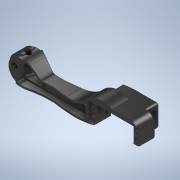
# Autodesk Inventor part: Perna_Esq_v2
Saved by Autodesk Inventor 2020 (Build 240168000, 168)
## iProperties
Created: 2021-05-05
Part Number: Perna_Esq_v2
Material: Plástico PC/ABS
Document SubType Name: Modeling
Designer: JCarlos
Density: 0.357273 g/cm^3
Appearance: Brilhosa - Preta
Mass: 11.0477 g
Surface Area: 184.649 cm^2
Volume: 30.9223 cm^3
Author: JCarlos
Autodesk Inventor part; units mm, degrees
sketch "Esboço1" plane through (0, 0, 0) normal (0, 0, 1) x (1, 0, 0)
  line L0 (97.4332, 6) -> (97.4332, -6)
  line L1 (16.7086, -15) -> (-37.5668, -15)
  line L2 (-37.286, -11) -> (-21.0787, -11)
  line L3 (-18.1298, -3.8807) -> (-30.0859, 8.0754)
  line L4 (-26.9602, 10.6066) -> (-17.8181, 1.4645)
  line L5 (-14.2825, 0) -> (14.2825, 0)
  arc A0 (67.4332, 15) -> (35.9332, 7.5) centre (56.0954, -7.2813) ccw
  arc A1 (14.2825, 0) -> (35.9332, 7.5) centre (14.2825, 35) ccw
  line L6 (67.4332, 15) -> (88.4332, 15)
  arc A2 (-26.9602, 10.6066) -> (-37.5668, -15) centre (-37.5668, 0) ccw
  arc A3 (-21.0787, -11) -> (-18.1298, -3.8807) centre (-21.0787, -6.8296) ccw
  line L7 (-35.0263, 6.9801) -> (-40.1051, -6.9739)
  circle A4 centre (-43.6748, 2.2231) radius 3.25
  arc A5 (-40.1051, -6.9739) -> (-37.286, -11) centre (-37.286, -8) ccw
  arc A6 (-30.0859, 8.0754) -> (-35.0263, 6.9801) centre (-32.2072, 5.9541) ccw
  arc A7 (-17.8181, 1.4645) -> (-14.2825, 0) centre (-14.2825, 5) ccw
  line L8 (88.4332, -11) -> (88.4332, 10)
  line L9 (88.4332, 10) -> (47.4332, 10)
  line L10 (47.4332, 10) -> (47.4332, -11)
  line L11 (88.4332, -11) -> (92.4332, -11)
  arc A8 (16.7086, -15) -> (47.4332, -11) centre (16.7086, 105) ccw
  line L12 (-52.5668, 15) -> (-22.3891, 15)
  line L13 (-37.5668, 0) -> (-45.4526, 2.8702)
  arc A9 (97.4332, 6) -> (88.4332, 15) centre (88.4332, 6) ccw
  arc A10 (92.4332, -11) -> (97.4332, -6) centre (92.4332, -6) ccw
  point P0 (0, 0)
  point P1 (97.4332, -11)
  point P2 (97.4332, 15)
  point P3 (0, 15)
  point P4 (-75, 0)
  point P5 (47.8453, 16.3182)
  point P6 (0, -15)
  point P7 (97.4332, 0)
  point P8 (0, 0)
  dimension "d8" = 4
  dimension "d9" = 15
  dimension "d10" = 30
  dimension "d11" = 22.5
  dimension "d12" = 61.5
  dimension "d13" = 25
  dimension "d14" = 70
  dimension "d15" = 4
  dimension "d22" = 15
  dimension "d29" = 15
  dimension "d31" = 6.5
  dimension "d32" = 6.5
  dimension "d33" = 3
  dimension "d34" = 70
  dimension "d36" = 22
  dimension "d38" = 135
  dimension "d39" = 5
  dimension "d40" = 26
  dimension "d41" = 5
  dimension "d42" = 9
  dimension "d43" = 41
  dimension "d45" = 150
  dimension "d47" = 120
  dimension "d49" = 9
  dimension "d50" = 5
  dimension "d76" = 7.7187
  dimension "d172" = 4
  constraints: 28 end point, 22 point on circle, 17 tangent, 11 centre point, 7 point on line, 5 perpendicular, 4 horizontal, 3 horizontal alignment, 2 midpoint, 2 parallel, 2 vertical alignment, 1 coincident, 1 equal radius, 1 vertical
  measures "d8" distance between parallel lines of L1 L2
  measures "d9" distance between parallel lines of L1 L5
  measures "d10" distance from line of L6.start L0
  measures "d11" distance from line of A0.end L1
  measures "d12" distance from line of A0.end L0
  measures "d13" radius of A0
  measures "d14" diameter of A1
  measures "d15" distance between parallel lines of L3 L4
  measures "d22" radius of A2
  measures "d29" distance edge to line of A2 L7
  measures "d31" diameter of A4
  measures "d32" distance from line of L7 A4.centre
  measures "d33" radius of A5
  measures "d34" angle of L2 L7
  measures "d38" angle of L5 L4
  measures "d39" radius of A7
  measures "d40" distance between parallel lines of L11 L6
  measures "d41" distance between parallel lines of L9 L6
  measures "d42" distance between parallel lines of L0 L8
  measures "d43" distance between parallel lines of L8 L10
  measures "d47" radius of A8
  measures "d49" radius of A9
  measures "d50" radius of A10
  measures "d76" distance edge to line of A0 L9
  measures "d172" distance from line of A8.start L11
extrude "Extrusão1" add sketch "Esboço1" along normal mid plane 20
sketch "Esboço3" plane through (0, 0, 10) normal (0, 0, 1) x (1, 0, 0)
  line L0 (14.2825, 0) -> (-14.2825, 0) projected
  arc A0 (14.2825, 0) -> (35.9332, 7.5) centre (14.2825, 35) ccw projected
  line L1 (47.4332, -11) -> (47.4332, 10) projected
  arc A1 (16.7086, -15) -> (47.4332, -11) centre (16.7086, 105) ccw projected
  line L2 (-37.5668, -15) -> (16.7086, -15) projected
  arc A2 (-17.8181, 1.4645) -> (-14.2825, 0) centre (-14.2825, 5) ccw projected
  line L3 (-17.8181, 1.4645) -> (-26.9602, 10.6066) projected
  line L4 (-40.1051, -6.9739) -> (-35.0263, 6.9801) projected
  arc A3 (67.4332, 15) -> (35.9332, 7.5) centre (56.0954, -7.2813) ccw projected
  arc A4 (-26.9602, 10.6066) -> (-37.5668, -15) centre (-37.5668, 0) ccw projected
  line L5 (37.4332, 0.4464) -> (37.4332, -8.6259)
  arc A5 (16.7086, -13) -> (34.8956, -11.59) centre (16.7086, 105) ccw
  line L6 (16.7086, -13) -> (-37.5668, -13)
  line L7 (-28.3744, 9.1924) -> (-19.2323, 0.0503)
  arc A6 (-19.2323, 0.0503) -> (-14.2825, -2) centre (-14.2825, 5) ccw
  line L8 (-14.2825, -2) -> (14.2825, -2)
  arc A7 (14.2825, -2) -> (32.9219, 3.0379) centre (14.2825, 35) ccw
  line L9 (-40.8295, -8.9641) -> (-34.3042, 8.9641)
  arc A8 (-28.3744, 9.1924) -> (-29.6606, 10.3194) centre (-37.5668, 0) ccw
  arc A9 (-38.1435, -12.9872) -> (-37.5668, -13) centre (-37.5668, 0) ccw
  arc A10 (-29.6606, 10.3194) -> (-34.3042, 8.9641) centre (-31.4851, 7.938) ccw
  arc A11 (-40.8295, -8.9641) -> (-38.1435, -12.9872) centre (-38.0104, -9.9902) ccw
  arc A12 (34.8956, -11.59) -> (37.4332, -8.6259) centre (34.4332, -8.6259) ccw
  arc A13 (37.4332, 0.4464) -> (32.9219, 3.0379) centre (34.4332, 0.4464) ccw
  point P0 (0, 0)
  point P1 (37.4332, -11.1658)
  point P2 (37.4332, 7.9578)
  point P3 (-42.0131, -12.216)
  point P4 (-33.1206, 12.216)
  point P5 (41.4288, 12.9645)
  point P6 (-35.0263, 6.9801)
  point P7 (37.4332, 6.1374)
  dimension "d53" = 2
  dimension "d54" = 3
  dimension "d55" = 2
  dimension "d56" = 10
  dimension "d58" = 3
  dimension "d59" = 2
  dimension "d60" = 2
  dimension "d74" = 3
  dimension "d75" = 2
  constraints: 23 point on circle, 10 end point, 9 centre point, 8 tangent, 5 point on line, 1 collinear, 1 equal radius, 3 other
  measures "d53" distance between parallel lines of L0 L8
  measures "d54" radius of A10
  measures "d55" distance between parallel lines of L2 L6
  measures "d56" distance between parallel lines of L1 L5
  measures "d58" radius of A12
  measures "d59" radial gap between concentric circles of A4 A8
  measures "d60" radial gap between concentric circles of A4 A9
  measures "d74" radius of A13
  measures "d75" radial gap between concentric circles of A0 A7
extrude "Extrusão2" cut sketch "Esboço3" against normal blind 8
sketch "Esboço4" plane through (0, 0, 10) normal (0, 0, 1) x (1, 0, 0)
  line L0 (-37.4284, 14.9994) -> (-38.161, 12.9864)
  line L1 (-40.8295, -8.9641) -> (-34.3042, 8.9641) projected
  line L2 (-46.3695, -9.5662) -> (-47.1022, -11.5792)
  arc A0 (-38.161, 12.9864) -> (-46.3695, -9.5662) centre (-37.5668, 0) ccw
  arc A1 (-37.4284, 14.9994) -> (-47.1022, -11.5792) centre (-37.5668, 0) ccw
  arc A2 (-26.9602, 10.6066) -> (-37.5668, -15) centre (-37.5668, 0) ccw projected
  point P0 (0, 0)
  dimension "d67" = 5
  dimension "d68" = 13
  constraints: 4 end point, 4 point on circle, 3 concentric, 2 centre point, 1 collinear
  measures "d67" distance between parallel lines of L1 L0
  measures "d68" radius of A0
extrude "Extrusão3" cut sketch "Esboço4" against normal blind 3
sketch "Esboço5" plane through (0, 0, 10) normal (0, 0, 1) x (1, 0, 0)
  line L0 (-37.4284, 14.9994) -> (-38.161, 12.9864) projected
  line L1 (-37.4284, 14.9994) -> (-38.161, 12.9864)
  line L2 (-40.8295, -8.9641) -> (-34.3042, 8.9641) projected
  line L3 (-33.1206, 12.216) -> (-32.4365, 14.0954)
  arc A0 (-26.9602, 10.6066) -> (-37.5668, -15) centre (-37.5668, 0) ccw projected
  line L4 (-47.1022, -11.5792) -> (-46.3695, -9.5662)
  line L5 (-42.0131, -12.216) -> (-42.6971, -14.0954)
  arc A1 (-47.1022, -11.5792) -> (-42.6971, -14.0954) centre (-37.5668, 0) ccw
  arc A2 (-32.4365, 14.0954) -> (-37.4284, 14.9994) centre (-37.5668, 0) ccw
  arc A3 (-38.161, 12.9864) -> (-46.3695, -9.5662) centre (-37.5668, 0) ccw projected
  arc A4 (-33.1206, 12.216) -> (-38.161, 12.9864) centre (-37.5668, 0) ccw
  arc A5 (-46.3695, -9.5662) -> (-42.0131, -12.216) centre (-37.5668, 0) ccw
  point P0 (0, 0)
  point P1 (-47.1022, -11.5792)
  point P2 (-42.6971, -14.0954)
  dimension "d187" = 13
  dimension "d188" = 13
  constraints: 9 point on circle, 8 end point, 4 centre point, 3 collinear, 1 coincident, 1 concentric, 1 parallel
  measures "d187" radius of A5
  measures "d188" radius of A4
extrude "Extrusão4" cut sketch "Esboço5" against normal through all contours A0 L3 A4 L0 | L4 A5 L5 A0
mirror "Espelhamento1" about plane through (0, 0, 0) normal (0, 0, 1) of "Extrusão2", "Extrusão3"
sketch "Esboço7" plane through (0, 0, -10) normal (0, 0, -1) x (-1, 0, 0)
  line L0 (-88.4332, 10) -> (-47.4332, 10) projected
  line L1 (-88.4332, 10) -> (-47.4332, 10)
  line L2 (-47.4332, 10) -> (-47.4332, 11.8053)
  line L3 (-64.6886, 15) -> (-85.4332, 15)
  line L4 (-88.4332, 12) -> (-88.4332, 10)
  line L5 (-47.4332, 10) -> (-47.4332, -11) projected
  arc A0 (-49.1218, 13.7809) -> (-64.6886, 15) centre (-64.6886, -85) ccw
  line L6 (-67.4332, 15) -> (-88.4332, 15) projected
  arc A1 (-85.4332, 15) -> (-88.4332, 12) centre (-85.4332, 12) ccw
  arc A2 (-47.4332, 11.8053) -> (-49.1218, 13.7809) centre (-49.4332, 11.8053) ccw
  point P0 (0, 0)
  point P1 (-47.4332, 13.5)
  point P2 (-47.4332, 10)
  dimension "d78" = 100
  dimension "d79" = 3.5
  dimension "d81" = 3
  dimension "d82" = 2
  constraints: 8 end point, 7 point on circle, 5 tangent, 3 centre point, 2 collinear, 2 parallel, 1 horizontal, 1 perpendicular, 1 point on line
  measures "d78" radius of A0
  measures "d79" distance of L1.end point (-47.433, 13.5)
  measures "d81" radius of A1
  measures "d82" radius of A2
extrude "Extrusão5" add sketch "Esboço7" along normal blind 13.5
sketch "Esboço8" plane through (0, 0, -23.5) normal (0, 0, -1) x (-1, 0, 0)
  line L0 (-47.4332, 10) -> (-47.4332, 11.8053) projected
  arc A0 (-47.4332, 11.8053) -> (-49.1218, 13.7809) centre (-49.4332, 11.8053) ccw projected
  arc A1 (-49.1218, 13.7809) -> (-64.6886, 15) centre (-64.6886, -85) ccw projected
  line L1 (-64.6886, 15) -> (-85.4332, 15) projected
  arc A2 (-85.4332, 15) -> (-88.4332, 12) centre (-85.4332, 12) ccw projected
  line L2 (-88.4332, 12) -> (-88.4332, 10) projected
  line L3 (-47.4332, 10) -> (-47.4332, -11) projected
  line L4 (-47.4332, 8.2125) -> (-47.4332, -7)
  line L5 (-51.4332, -11) -> (-84.4332, -11)
  line L6 (-88.4332, -7) -> (-88.4332, 10)
  line L7 (-92.4332, -11) -> (-88.4332, -11) projected
  arc A3 (-88.4332, -7) -> (-84.4332, -11) centre (-84.4332, -7) ccw
  arc A4 (-51.4332, -11) -> (-47.4332, -7) centre (-51.4332, -7) ccw
  point P0 (0, 0)
  point P1 (-47.4332, -11)
  point P2 (-88.4332, -11)
  point P3 (-47.4332, -7)
  dimension "d88" = 4
  constraints: 6 end point, 5 centre point, 5 point on line, 4 point on circle, 4 tangent, 1 collinear, 1 equal radius, 1 parallel, 1 perpendicular
  measures "d88" radius of A3
extrude "Extrusão6" add sketch "Esboço8" against normal blind 3
sketch "Esboço11" plane through (-37.5668, -15, 10) normal (0, -1, 0) x (1, 0, 0)
  line L0 (0.1384, -17) -> (-15, -17) projected
  arc A0 (35.74, -16.5162) -> (5, -20) centre (33.7706, -136.5) ccw
  line L1 (61.3045, -10) -> (-29.1591, -10)
  line L2 (0, 0) -> (54.2754, 0) projected
  line L3 (-13, -20) -> (-0.5942, -20) projected
  line L4 (54.2754, -20) -> (85, -20) projected
  line L5 (85, -20) -> (5, -20)
  arc A1 (35.74, -16.5162) -> (85, -20) centre (85, 330) ccw
  line L6 (54.2754, -20) -> (0, -20) projected
  point P0 (37.5668, -10)
  point P1 (-9.5354, -17)
  point P2 (-8.8027, -20)
  point P3 (4.4463, -20)
  point P4 (-4.4463, -20)
  dimension "d96" = 10
  dimension "d97" = 13
  dimension "d98" = 350
  dimension "d99" = 120
  dimension "d101" = 20
  constraints: 5 end point, 4 point on circle, 2 centre point, 1 collinear, 1 horizontal, 1 tangent
  measures "d96" distance between parallel lines of L2 L1
  measures "d98" radius of A1
  measures "d99" radius of A0
  measures "d101" horizontal distance of L0.end L5.end
extrude "Extrusão9" cut sketch "Esboço11" against normal through all
mirror "Espelhamento2" about plane through (0, 0, 0) normal (0, 0, 1) of "Extrusão9"
ref_plane "Plano de trabalho4" through (-48.1734, -10.6066, 0) normal (-0.7071068, -0.7071068, 0) x (0.7071068, -0.7071068, 0)
ref_plane "Plano de trabalho6" through (67.9332, -11, 10) normal (-1, 0, 0) x (0, 0, 1)
sketch "Esboço19" plane through (0, 0, 10) normal (0, 0, 1) x (1, 0, 0)
  line L0 (92.4332, 9.5061) -> (92.4332, -9.398)
  line L1 (67.9332, -38.8118) -> (67.9332, 27.1405) projected
  line L2 (93.7884, -5.5) -> (90.981, -5.5)
  line L3 (93.7884, 4.5) -> (90.981, 4.5)
  line L4 (88.4332, -11) -> (92.4332, -11) projected
  circle A0 centre (92.4332, 4.5) radius 1.75
  circle A1 centre (92.4332, -5.5) radius 1.75
  line L5 (47.4332, 10) -> (88.4332, 10) projected
  point P0 (0, 0)
  dimension "d152" = 24.5
  dimension "d153" = 10
  dimension "d155" = 3.5
  dimension "d156" = 3.5
  dimension "d161" = 5.5
  constraints: 6 end point, 4 point on line, 2 centre point, 2 vertical alignment, 1 horizontal, 1 parallel, 1 vertical
  measures "d152" distance between parallel lines of L1 L0
  measures "d153" distance between parallel lines of L2 L3
  measures "d155" diameter of A0
  measures "d156" diameter of A1
  measures "d161" distance between parallel lines of L3 L5
extrude "Furos_Fix_Motor" cut sketch "Esboço19" against normal blind 19
sketch "Esboço16" plane through (88.4332, -11, 10) normal (-1, 0, 0) x (0, 0, 1)
  line L0 (-13.3, 8.35) -> (-16, 8.35)
  line L1 (-16, 8.35) -> (-16, 2.65)
  line L2 (-16, 2.65) -> (-13.3, 2.65)
  line L3 (-13.3, 2.65) -> (-13.3, 8.35)
  line L4 (0, 21) -> (0, 0) projected
  line L5 (-13.3, 5.5) -> (-16, 5.5)
  line L6 (-20, 0) -> (0, 0) projected
  line L7 (-13.3, 18.35) -> (-16, 18.35)
  line L8 (-16, 18.35) -> (-16, 12.65)
  line L9 (-16, 12.65) -> (-13.3, 12.65)
  line L10 (-13.3, 12.65) -> (-13.3, 18.35)
  line L11 (-13.3, 15.5) -> (-16, 15.5)
  point P0 (-10, 11)
  point P1 (-15, 0)
  point P2 (-9, 11.5)
  dimension "d141" = 2.7
  dimension "d142" = 5.7
  dimension "d143" = 16
  dimension "d145" = 2.7
  dimension "d146" = 5.7
  dimension "d147" = 10
  dimension "d170" = 5.5
  constraints: 20 end point, 4 midpoint, 4 parallel, 2 horizontal, 2 perpendicular, 1 collinear
  measures "d141" distance of L1.end L2.end
  measures "d142" distance of L2.end L0.start
  measures "d143" distance between parallel lines of L1 L4
  measures "d145" distance of L8.end L9.end
  measures "d146" distance of L9.end L7.start
  measures "d147" distance between parallel lines of L11 L5
  measures "d170" distance from line of L4.start L11
extrude "Encaixe_Porcas" cut sketch "Esboço16" against normal blind 7.5
mirror "Espelhamento5" about plane through (67.9332, -11, 10) normal (-1, 0, 0) of "Encaixe_Porcas", "Furos_Fix_Motor"
sketch "Esboço9" plane through (0, 0, -23.5) normal (0, 0, -1) x (-1, 0, 0)
  circle A0 centre (-77.9332, -0.5) radius 2.425
  line L0 (-88.4332, 12) -> (-88.4332, -7) projected
  line L1 (-84.4332, -11) -> (-51.4332, -11) projected
  circle A1 centre (-92.4332, -5.5) radius 1.75 projected
  point P0 (0, 0)
  dimension "d89" = 4.85
  dimension "d159" = 14.5
  dimension "d171" = 5
  constraints: 1 centre point
  measures "d89" diameter of A0
  measures "d159" horizontal distance of A1.centre A0.centre
  measures "d171" vertical distance of A1.centre A0.centre
extrude "Pino_Eixo" add sketch "Esboço9" along normal blind 7 contours A0
fillet "Arredondamento1" radius 1.5 9 edges at (48.6048, -9.8284, -23.5) (47.4332, 2.4027, -23.5) (47.9129, 13.1048, -23.5) (56.8814, 14.6948, -23.5) (75.0609, 15, -23.5) (87.5545, 14.1213, -23.5) (88.4332, 2.5, -23.5) (87.2616, -9.8284, -23.5) (67.9332, -11, -23.5)
chamfer "Chanfro1" distance 0.5 angle 45 1 edges at (80.3582, -0.5, -30.5)
sketch "Esboço20" plane through (0, 0, 10) normal (0, 0, 1) x (1, 0, 0)
  line L0 (96.4954, 10) -> (41.4332, 10)
  line L1 (40.4332, 9) -> (40.4332, -10)
  line L2 (41.4332, -11) -> (97.4332, -11)
  line L3 (97.4332, -11) -> (97.4332, 6)
  arc A0 (97.4332, 6) -> (88.4332, 15) centre (88.4332, 6) ccw projected
  line L4 (97.4332, -6) -> (97.4332, 6) projected
  arc A1 (92.4332, -11) -> (97.4332, -6) centre (92.4332, -6) ccw projected
  line L5 (47.4332, 10) -> (88.4332, 10) projected
  circle A2 centre (43.4332, 4.5) radius 1.75 projected
  arc A3 (41.4332, 10) -> (40.4332, 9) centre (41.4332, 9) ccw
  arc A4 (40.4332, -10) -> (41.4332, -11) centre (41.4332, -10) ccw
  point P0 (0, 0)
  dimension "d165" = 3
  dimension "d166" = 1
  dimension "d167" = 21
  constraints: 8 end point, 6 point on circle, 4 tangent, 2 centre point, 2 collinear, 2 parallel, 1 equal radius, 1 horizontal, 1 perpendicular, 1 other
  measures "d165" distance from line of A2.centre L1
  measures "d166" radius of A3
  measures "d167" distance between parallel lines of L5 L2
extrude "Extrusão13" cut sketch "Esboço20" against normal blind 3.5
fillet "Arredondamento2" radius 1 1 edges at (80.3582, -0.5, -23.5)
fillet "Arredondamento3" radius 1 21 edges at (95.9687, -9.5355, 6.5) (90.4332, -11, 6.5) (97.1956, 8.0542, 6.5) (97.4332, 0, 6.5) (44.4331, 10, 9.9871) (40.691, 9.6702, 9.9351) (40.4332, -0.5, 9.93) (40.6903, -10.6694, 9.935) (44.4331, -11, 9.9871) (71.9643, 10, 10) (96.4954, 10, 8.25) (97.4332, 0, -10) (95.9687, -9.5355, -10) (90.4332, -11, -10) (86.9332, 15, -10) (94.7971, 12.364, -10) (88.4332, -11, -1.75) (88.4332, -0.5, 6.5) (88.4332, -0.5, -10) (47.4332, -0.5, 6.5) (47.4332, -0.5, -10)
sketch "Esboço23" plane through (-48.1734, -10.6066, 0) normal (-0.7071068, -0.7071068, 0) x (0.7071068, -0.7071068, 0)
  circle A0 centre (0.4452, 0) radius 3
  line L0 (1.4452, -7) -> (1.4452, 7) projected
  line L1 (-15, 7) -> (1.4452, 7) projected
  point P0 (26.5638, 0)
  point P1 (1.4452, -3)
  point P2 (-10.5083, 7)
  dimension "d189" = 6
  dimension "d190" = 1
  dimension "d191" = 7
  constraints: 1 centre point
  measures "d189" diameter of A0
  measures "d190" distance from line of A0.centre L0
  measures "d191" distance from line of L1 A0.centre
extrude "Extrusão14" cut sketch "Esboço23" against normal blind 6.5
ref_plane "Plano de trabalho7" through (-43.6748, 2.2231, 10) normal (-0.3420201, -0.9396926, 0) x (0.9396926, -0.3420201, 0)
chamfer "Chanfro2" distance 2.5 angle 30 2 edges at (95.9332, -2.65, -4.65) (95.9332, -8.35, -4.65) measured on face at (95.9332, -7.85, -4.65) measured on face at (95.9332, -3.15, -4.65)
chamfer "Chanfro3" distance 2.5 angle 30 2 edges at (95.9332, 7.35, -4.65) (95.9332, 1.65, -4.65) measured on face at (95.9332, 6.85, -4.65) measured on face at (95.9332, 2.15, -4.65)
chamfer "Chanfro4" distance 2.5 angle 30 2 edges at (39.9332, -2.65, -4.65) (39.9332, -8.35, -4.65) measured on face at (39.9332, -7.85, -4.65) measured on face at (39.9332, -3.15, -4.65)
chamfer "Chanfro5" distance 2.5 angle 30 2 edges at (39.9332, 1.65, -4.65) (39.9332, 7.35, -4.65) measured on face at (39.9332, 2.15, -4.65) measured on face at (39.9332, 6.85, -4.65)
mirror "Espelhamento7" about plane through (-43.6748, 2.2231, 10) normal (-0.3420201, -0.9396926, 0) of "Extrusão14"
equation "\"d55\" = d53"
equation "\"d59\" = d53"
equation "\"d60\" = d55"
equation "\"d75\" = d53"
